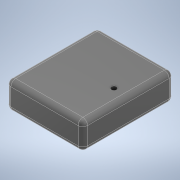
# Autodesk Inventor part: batterybox
Saved by Autodesk Inventor 2022 (Build 260153000, 153)
## iProperties
Created: 2022-04-20
Part Number: batterybox
Material: ABS プラスチック
Document SubType Name: Modeling
Designer: Yazawa
Density: 1.06 g/cm^3
Appearance: 滑らか - 黒
Author: Yazawa
Autodesk Inventor part; units mm, degrees
ref_plane "YZ Plane" through (0, 0, 0) normal (1, 0, 0) x (0, 1, 0)
ref_plane "XZ Plane" through (0, 0, 0) normal (0, 1, 0) x (-1, 0, 0)
ref_plane "XY Plane" through (0, 0, 0) normal (0, 0, 1) x (1, 0, 0)
sketch "スケッチ1" plane through (0, 0, 0) normal (0, 1, 0) x (-1, 0, 0)
  line L0 (20.1905, 18.381) -> (-27.8095, 18.381)
  line L1 (-27.8095, 18.381) -> (-27.8095, -38.619)
  line L2 (-27.8095, -38.619) -> (20.1905, -38.619)
  line L3 (20.1905, -38.619) -> (20.1905, 18.381)
  point P0 (0, 0)
  dimension "d0" = 48
  dimension "d1" = 57
  constraints: 8 end point, 2 parallel, 1 horizontal, 1 perpendicular
  measures "d0" distance of L1.end L2.end
  measures "d1" distance of L0.end L1.end
extrude "押し出し1" add sketch "スケッチ1" along normal blind 17
fillet "フィレット1" radius 3 12 edges at (27.8095, 17, -10.119) (3.8095, 17, -38.619) (-20.1905, 17, -10.119) (3.8095, 17, 18.381) (-20.1905, 8.5, 18.381) (27.8095, 8.5, 18.381) (3.8095, 0, 18.381) (27.8095, 0, -10.119) (-20.1905, 0, -10.119) (-20.1905, 8.5, -38.619) (27.8095, 8.5, -38.619) (3.8095, 0, -38.619)
sketch "スケッチ2" plane through (0, 17, 0) normal (0, 1, 0) x (1, 0, 0)
  line L0 (18.8095, 10.119) -> (18.8095, 38.619) construction
  line L1 (-17.1905, 38.619) -> (24.8095, 38.619) construction
  line L2 (18.8095, 10.119) -> (18.8095, -18.381) construction
  line L3 (24.8095, -18.381) -> (-17.1905, -18.381) construction
  line L4 (27.8095, -15.381) -> (27.8095, 35.619) construction
  point P0 (0, 0)
  dimension "d5" = 9
  constraints: 4 end point, 3 point on line, 1 collinear, 1 vertical
  measures "d5" distance from line of L4 L0.start
hole "穴1" at (18.8095, 17, -10.119) direction (0, -1, 0) diameter 3.4 depth 17 clearance for "Countersunk Flat Head Screw ISO 2009/7046" size "M3" standard "ISO"
